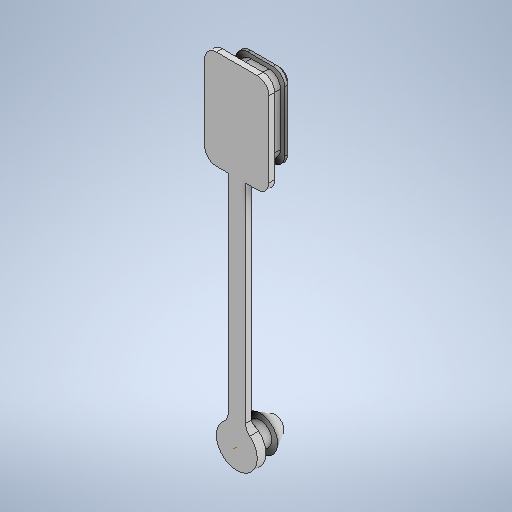
# Autodesk Inventor part: USB-C_cover
Saved by Autodesk Inventor 2025.2 (Build 292293000, 293)
## iProperties
Created: 2024-11-18
Part Number: USB-C_cover
Material: Generic
Document SubType Name: Modeling
Designer: matss
Density: 1 g/cm^3
Appearance: Default
Author: matss
Autodesk Inventor part; units mm, degrees
ref_plane "YZ Plane" through (0, 0, 0) normal (1, 0, 0) x (0, 1, 0)
ref_plane "XZ Plane" through (0, 0, 0) normal (0, 1, 0) x (-1, 0, 0)
ref_plane "XY Plane" through (0, 0, 0) normal (0, 0, 1) x (1, 0, 0)
sketch "Sketch1" plane through (0, 0, 0) normal (0, 1, 0) x (-1, 0, 0)
  line L0 (0, 0) -> (3.5, 0)
  line L1 (3.5, 0) -> (3.5, -1.5)
  line L2 (3.5, -1.5) -> (2, -1.5)
  line L3 (2, -1.5) -> (2, -4)
  line L4 (2, -4) -> (3, -4)
  line L5 (3, -4) -> (1.5, -6.5981)
  line L6 (1.5, -6.5981) -> (0, -6.5981)
  line L7 (0, -6.5981) -> (0, 0)
  line L8 (0, -7.9177) -> (0, 1.3196) projected
  dimension "d0" = 3.5
  dimension "d1" = 1.5
  dimension "d3" = 2.5
  dimension "d4" = 2
  dimension "d5" = 1
  dimension "d6" = 1.5
  dimension "d7" = 60
  constraints: 16 end point, 4 perpendicular, 3 horizontal
  measures "d0" distance of L0.start L0.end
  measures "d1" distance of L0.end L1.end
  measures "d3" distance of L2.end L3.end
  measures "d4" distance from line of L0.start L3
  measures "d5" distance of L3.end L4.end
  measures "d6" horizontal distance of L0.start L5.end
  measures "d7" angle of L4 L5
revolve "Revolution1" add sketch "Sketch1" angle 360 about axis through (0, 0, -10) along (0, 0, 1)
sketch "Sketch2" plane through (0, 0, 0) normal (0, 0, 1) x (1, 0, 0)
  circle A0 centre (0, 0) radius 3.5 construction
  line L0 (-1.5, 0) -> (1.5, 0)
  line L1 (1.5, 0) -> (1.5, 40)
  line L2 (1.5, 40) -> (-1.5, 40)
  line L3 (-1.5, 40) -> (-1.5, 0)
  line L4 (-5.5, 40) -> (5.5, 40)
  line L5 (5.5, 40) -> (5.5, 57)
  line L6 (5.5, 57) -> (-5.5, 57)
  line L7 (-5.5, 57) -> (-5.5, 40)
  point P0 (0, 40)
  dimension "d9" = 3
  dimension "d10" = 40
  dimension "d11" = 11
  dimension "d12" = 17
  constraints: 16 end point, 4 parallel, 3 midpoint, 2 horizontal, 2 perpendicular, 1 coincident
  measures "d9" distance of L2.end L1.end
  measures "d10" distance of L0.end L1.end
  measures "d11" distance of L6.end L5.end
  measures "d12" distance of L5.end L4.end
extrude "Extrusion1" add sketch "Sketch2" against normal blind 1
sketch "Sketch3" plane through (0, 0, -1) normal (0, 0, -1) x (-1, 0, 0)
  line L0 (3.5, 55) -> (-3.5, 55)
  line L1 (-3.5, 55) -> (-3.5, 42)
  line L2 (-3.5, 42) -> (3.5, 42)
  line L3 (3.5, 42) -> (3.5, 55)
  line L4 (5.5, 57) -> (-5.5, 57) projected
  line L5 (5.5, 40) -> (5.5, 57) projected
  point P0 (0, 0)
  point P1 (0, 55)
  point P2 (0, 57)
  point P3 (3.5, 48.5)
  point P4 (5.5, 48.5)
  dimension "d15" = 7
  dimension "d16" = 13
  constraints: 8 end point, 4 midpoint, 2 parallel, 1 horizontal, 1 horizontal alignment, 1 perpendicular, 1 vertical alignment
  measures "d15" distance of L2.end L1.end
  measures "d16" distance of L1.end L0.end
extrude "Extrusion2" add sketch "Sketch3" along normal blind 3
sketch "Sketch4" plane through (0, 0, -4) normal (0, 0, -1) x (-1, 0, 0)
  line L0 (-3.5, 55) -> (-3.5, 42) projected
  line L1 (-3.5, 42) -> (3.5, 42) projected
  line L2 (3.5, 42) -> (3.5, 55) projected
  line L3 (3.5, 55) -> (-3.5, 55) projected
  line L4 (4.2, 55.7) -> (4.2, 41.3)
  line L5 (4.2, 41.3) -> (-4.2, 41.3)
  line L6 (-4.2, 41.3) -> (-4.2, 55.7)
  line L7 (-4.2, 55.7) -> (4.2, 55.7)
  point P0 (0, 0)
  dimension "d20" = 0.7
  constraints: 8 end point, 3 other
  measures "d20" distance between parallel lines of L2 L4
extrude "Extrusion3" add sketch "Sketch4" along normal blind 1 contours L3 L2 L1 L0 | L4 L5 L6 L7
fillet "Fillet1" radius 2 12 edges at (-5.5, 57, -0.5) (-5.5, 40, -0.5) (5.5, 57, -0.5) (5.5, 40, -0.5) (3.5, 42, -2.5) (3.5, 55, -2.5) (-3.5, 55, -2.5) (-3.5, 42, -2.5) (-4.2, 41.3, -4.5) (4.2, 41.3, -4.5) (4.2, 55.7, -4.5) (-4.2, 55.7, -4.5)
chamfer "Chamfer1" distance 0.5 angle 45 8 edges at (-4.2, 48.5, -5) (-3.6142, 55.1142, -5) (0, 55.7, -5) (3.6142, 55.1142, -5) (4.2, 48.5, -5) (3.6142, 41.8858, -5) (0, 41.3, -5) (-3.6142, 41.8858, -5)
fillet "Fillet2" radius 2 3 edges at (1.5, 3.1623, -0.5) (0, 3.5, -1) (-1.5, 3.1623, -0.5)
body "Solid1"
